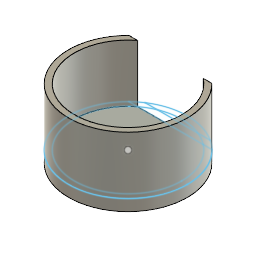
motor_base (Autodesk Fusion 360 design; units mm, degrees)
part number: 2025-11-06-14-13-39-273
Autodesk Fusion 360 part; units mm, degrees
sketch "Sketch1" plane through (0, 0, 0) normal (0, 1, 0) x (1, 0, 0)
  circle A0 centre (26.358, -28.2925) radius 15.5
  line L0 (17.858, -15.331) -> (34.858, -15.331)
  circle A1 centre (26.358, -28.2925) radius 14
  line L1 (17.8035, -17.2101) -> (34.9126, -17.2101)
  line L2 (34.9126, -17.2101) -> (37.1946, -17.2101)
  line L3 (17.8035, -17.2101) -> (15.5215, -17.2101)
  dimension "d1" = 31
  dimension "d2" = 17
  dimension "d3" = 28
  constraint coincident A0 L0.start
  constraint coincident A0 L0.end
  constraint horizontal L0
  constraint concentric A0 A1
  constraint coincident A1 L1.start
  constraint horizontal L1
  constraint coincident A1 L1.end
  constraint coincident A0 L2.end
  constraint parallel L1 L2
  constraint coincident A0 L3.end
  constraint parallel L1 L3
  measures "d1" diameter of A0
  measures "d2" distance of L0.start L0.end
  measures "d3" diameter of A1
extrude "Extrude1" add sketch "Sketch1" along normal blind 15 contours A0 A1 L2 L3 makes body 1
extrude "Extrude2" add sketch "Sketch1" against normal blind 3 contours A0 A1 L2 L3 bodies 1
extrude "Extrude3" add sketch "Sketch1" against normal blind 3 contours A1 L1 bodies 1
sketch "Sketch2" plane through (0, 0, 0) normal (0, 1, 0) x (1, 0, 0)
  circle A0 centre (26.3651, -28.3162) radius 3.5
  dimension "d11" = 7
  measures "d11" diameter of A0
extrude "Extrude4" add sketch "Sketch2" against normal blind 5 separate body makes body 2
combine "Combine1" operation add target body 2 tool bodies 1
